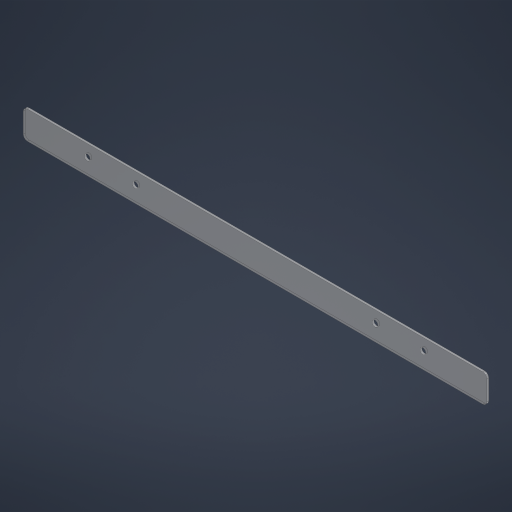
# Autodesk Inventor part: wedge
Saved by Autodesk Inventor 2024 (Build 280153000, 153)
## iProperties
Created: 2023-11-18
Part Number: wedge
Material: Polycarbonate, Clear
Document SubType Name: Modeling
Designer: macbook
Density: 1.2 g/cm^3
Appearance: Polycarbonate - Clear(1)
Author: macbook
Autodesk Inventor part; units mm, degrees
ref_plane "YZ Plane" through (0, 0, 0) normal (1, 0, 0) x (0, 1, 0)
ref_plane "XZ Plane" through (0, 0, 0) normal (0, 1, 0) x (-1, 0, 0)
ref_plane "XY Plane" through (0, 0, 0) normal (0, 0, 1) x (1, 0, 0)
sketch "Sketch1" plane through (0, 0, 0) normal (0, 0, 1) x (1, 0, 0)
  line L0 (-374.65, -3.175) -> (-374.65, 38.1)
  line L1 (-371.475, 50.8) -> (-9.525, 50.8)
  line L2 (-6.35, 38.1) -> (-6.35, 22.225)
  arc A0 (-371.475, 50.8) -> (-374.65, 47.625) centre (-371.475, 47.625) ccw
  arc A1 (-6.35, 47.625) -> (-9.525, 50.8) centre (-9.525, 47.625) ccw
  line L3 (-374.65, 50.8) -> (-374.65, 41.275)
  line L4 (-371.475, 41.275) -> (-9.525, 41.275)
  arc A2 (-371.475, 41.275) -> (-374.65, 38.1) centre (-371.475, 38.1) ccw
  arc A3 (-6.35, 38.1) -> (-9.525, 41.275) centre (-9.525, 38.1) ccw
  line L5 (-374.65, 41.275) -> (-374.65, 22.225)
  line L6 (-371.475, 19.05) -> (-9.525, 19.05)
  arc A4 (-374.65, 22.225) -> (-371.475, 19.05) centre (-371.475, 22.225) ccw
  arc A5 (-9.525, 19.05) -> (-6.35, 22.225) centre (-9.525, 22.225) ccw
  point P0 (-6.35, 50.8)
  point P1 (-6.35, 41.275)
  point P2 (-374.65, 19.05)
  point P3 (-6.35, 19.05)
  point P4 (-374.65, 22.225)
  dimension "d25" = 9.525
  dimension "d26" = 3.175
  dimension "d27" = 22.225
  dimension "d28" = 3.175
  dimension "d29" = 361.95
  constraints: 15 point on line, 14 end point, 12 point on circle, 12 tangent, 6 centre point, 4 perpendicular, 3 equal radius, 2 vertical
  measures "d25" distance of L3.start L3.end
  measures "d26" radius of A2
  measures "d27" distance of L3.end point (-374.65, 19.05)
  measures "d28" radius of A4
  measures "d29" distance of L1.start L1.end
extrude "Extrusion1" add sketch "Sketch1" along normal blind 1.5875
sketch "Sketch2" plane through (0, 0, 1.5875) normal (0, 0, 1) x (1, 0, 0)
  line L0 (-381, 50.8) -> (-323.85, 50.8)
  line L1 (-323.85, 50.8) -> (-273.05, 50.8)
  line L2 (-381, 0) -> (-330.2, 0)
  line L3 (-323.85, 50.8) -> (-323.85, 31.75)
  line L4 (0, 50.8) -> (-57.15, 50.8)
  line L5 (-57.15, 50.8) -> (-107.95, 50.8)
  line L6 (0, 0) -> (-50.8, 0)
  line L7 (-57.15, 50.8) -> (-57.15, 31.75)
  line L8 (-273.05, 50.8) -> (-285.75, 50.8)
  line L9 (-3.175, 50.8) -> (-377.825, 50.8) projected
  line L10 (-285.75, 50.8) -> (-285.75, 31.75)
  line L11 (-107.95, 50.8) -> (-95.25, 50.8)
  line L12 (-95.25, 50.8) -> (-95.25, 31.75)
  line L13 (0, 50.8) -> (0, 41.275)
  line L14 (0, -3.175) -> (0, 47.625) projected
  line L15 (-374.65, 38.1) -> (-374.65, 22.225) projected
  line L16 (-381, 41.275) -> (0, 41.275)
  point P0 (-381, 47.625)
  point P1 (-381, -3.175)
  point P2 (-381, 19.05)
  dimension "d4" = 57.15
  dimension "d5" = 50.8
  dimension "d21" = 12.7
  dimension "d22" = 12.7
  dimension "d24" = 9.525
  constraints: 28 end point, 4 coincident, 3 perpendicular, 3 point on line, 1 horizontal, 1 vertical, 2 other
  measures "d4" distance of L0.start L0.end
  measures "d5" distance of L0.end L1.end
  measures "d21" distance of L1.end L8.end
  measures "d22" distance of L5.end L11.end
  measures "d24" distance of L4.start L13.end
hole "Hole1" at (-323.85, 31.75, 1.5875) at (-57.15, 31.75, 1.5875) at (-285.75, 31.75, 1.5875) at (-95.25, 31.75, 1.5875) direction (0, 0, -1) diameter 4.7625 end through all
body "Solid1"
